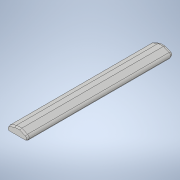
# Autodesk Inventor part: MINI-rail-spoolholder
Saved by Autodesk Inventor 2021 (Build 250183000, 183)
## iProperties
Created: 2019-06-28
Material: Všeobecné
Document SubType Name: Modeling
Density: 1 g/cm^3
Appearance: Výchozí
Project: ORIGINAL PRUSA MINI
Authority: Ing. Robert Turinský
Company: Prusa Development a.s.
Author: Ing. Robert Turinský
Title: MINI-rail-spoolholder
Revision Number: R4
Autodesk Inventor part; units mm, degrees
ref_plane "YZ Plane" through (0, 0, 0) normal (1, 0, 0) x (0, 1, 0)
ref_plane "XZ Plane" through (0, 0, 0) normal (0, 1, 0) x (-1, 0, 0)
ref_plane "XY Plane" through (0, 0, 0) normal (0, 0, 1) x (1, 0, 0)
sketch "Náčrt1" plane through (0, 0, 0) normal (0, 0, 1) x (1, 0, 0)
  line L0 (-5.05, 0) -> (5.05, 0)
  line L1 (0, -1.329763) -> (0, 6.054961)
  line L2 (-9.941711, 0) -> (9.941711, 0)
  line L3 (-5.719696, 3.366789) -> (-1.776776, 5)
  line L4 (-1.776776, 5) -> (1.776776, 5)
  line L5 (1.776776, 5) -> (5.719696, 3.366789)
  arc A0 (-5.719696, 3.366789) -> (-5.05, 0) centre (-5.05, 1.75) ccw
  arc A1 (5.05, 0) -> (5.719696, 3.366789) centre (5.05, 1.75) ccw
  line L6 (6.565544, 0.875) -> (6.060363, 0)
  line L7 (6.060363, 0) -> (5.05, 0)
  arc A2 (5.05, 0) -> (6.565544, 0.875) centre (5.05, 1.75) ccw
  line L8 (-5.05, 0) -> (-6.060363, 0)
  line L9 (-6.060363, 0) -> (-6.565544, 0.875)
  arc A3 (-6.565544, 0.875) -> (-5.05, 0) centre (-5.05, 1.75) ccw
  point P0 (0, 0)
  dimension "d0" = 135
  dimension "d1" = 1.75
  dimension "d2" = 13.6
  dimension "d3" = 5
  dimension "d12" = 60
  constraints: 16 end point, 10 point on circle, 9 tangent, 4 centre point, 2 collinear, 2 concentric, 2 horizontal, 2 point on line, 1 equal length, 1 symmetric about line, 1 other
  measures "d0" angle of L5 L3
  measures "d1" radius of A0
  measures "d3" distance between parallel lines of L0 L4
  measures "d12" angle of L2 L6
extrude "Vysunutí1" add sketch "Náčrt1" along normal blind 100
chamfer "Zkosení1" distance 0.5 angle 70 6 edges at (3.7482, 4.1834, 100) (6.7071, 2.3125, 100) (0, 0, 100) (-6.7071, 2.3125, 100) (-3.7482, 4.1834, 100) (0, 5, 100) measured on face at (0.5923, 1.6667, 100)
chamfer "Zkosení2" distance 0.5 angle 70 6 edges at (0, 0, 0) (6.7071, 2.3125, 0) (3.7482, 4.1834, 0) (-6.7071, 2.3125, 0) (-3.7482, 4.1834, 0) (0, 5, 0) measured on face at (0.5923, 1.6667, 0)
sketch "Náčrt2" plane through (-6.060363, 0, 98.626261) normal (0, -1, 0) x (1, 0, 0)
  line L0 (6.060363, -118.626261) -> (6.060363, 21.373739)
  line L1 (-3.459637, -98.626261) -> (15.580363, -98.626261)
  line L2 (12.120726, -97.252523) -> (0, -97.252523)
  line L3 (12.120726, -97.252523) -> (12.120726, 0)
  line L4 (0, 0) -> (12.120726, 0)
  line L5 (0, -97.252523) -> (0, 0)
  line L6 (7.435363, -6.126261) -> (4.685363, -6.126261)
  line L7 (4.685363, -6.126261) -> (4.685363, -91.126261)
  line L8 (4.685363, -91.126261) -> (7.435363, -91.126261)
  line L9 (7.435363, -91.126261) -> (7.435363, -6.126261)
  line L10 (11.832051, 1.373739) -> (0.288675, 1.373739)
  point P0 (6.060363, -98.626261)
  dimension "d13" = 2.75
  dimension "d14" = 7.5
  dimension "d15" = 7.5
  constraints: 8 end point, 2 parallel, 1 horizontal, 1 perpendicular, 1 other
  measures "d13" distance between parallel lines of L7 L9
  measures "d14" distance between parallel lines of L10 L6
  measures "d15" distance between parallel lines of L1 L8
extrude "Vysunutí2" cut sketch "Náčrt2" against normal blind 2.5 contours L8 L7 L6 L0 | L0 L6 L9 L8
equation "\"d9\" = d6"
equation "\"d11\" = d8"
equation "\"d15\" = d14"
equation "\"d6\" = 0.5"
equation "\"d8\" = 70deg"
